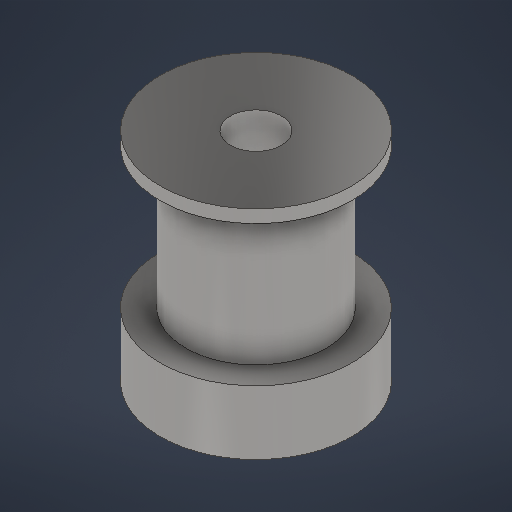
# Autodesk Inventor part: Timing belt pulley
Saved by Autodesk Inventor 2026.1 (Build 301233000, 233)
## iProperties
Created: 2025-02-25
Part Number: Timing belt pulley
Material: Generisch
Document SubType Name: Modeling
Designer: Luka Steib
Density: 1 g/cm^3
Appearance: Stahl - poliert
Author: Luka Steib
Autodesk Inventor part; units mm, degrees
ref_plane "YZ Plane" through (0, 0, 0) normal (1, 0, 0) x (0, 1, 0)
ref_plane "XZ Plane" through (0, 0, 0) normal (0, 1, 0) x (-1, 0, 0)
ref_plane "XY Plane" through (0, 0, 0) normal (0, 0, 1) x (1, 0, 0)
sketch "Skizze1" plane through (0, 0, 0) normal (0, 0, 1) x (1, 0, 0)
  circle A0 centre (0, 0) radius 7.5
  circle A1 centre (0, 0) radius 5.5
  circle A2 centre (0, 0) radius 2
  dimension "d0" = 15
  dimension "d3" = 11
  dimension "d9" = 4
  constraints: 3 centre point, 3 coincident
  measures "d0" diameter of A0
  measures "d3" diameter of A1
  measures "d9" diameter of A2
extrude "Extrusion2" add sketch "Skizze1" against normal blind 11 contours A1 | A2
sketch "Skizze2" plane through (0, 0, -11) normal (0, 0, -1) x (-1, 0, 0)
  circle A0 centre (0, 0) radius 7.5
  dimension "d6" = 15
  constraints: 1 centre point, 1 coincident
  measures "d6" diameter of A0
extrude "Extrusion3" add sketch "Skizze2" along normal blind 5
extrude "Extrusion4" cut sketch "Skizze1" along normal mid plane 50 contours A2
extrude "Extrusion5" add sketch "Skizze1" along normal blind 1 contours A0 | A1
